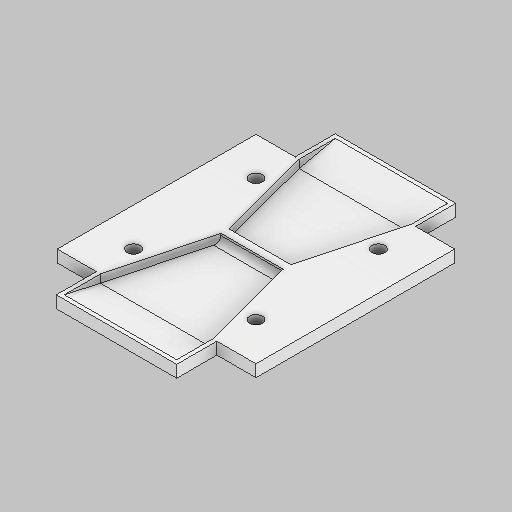
# Autodesk Inventor part: Part4
Saved by Autodesk Inventor 2025.2 (Build 292293000, 293)
## iProperties
Created: 2025-03-19
Part Number: Part4
Material: PC/ABS Plastic
Document SubType Name: Modeling
Designer: joaki
Density: 1.1 g/cm^3
Appearance: Smooth - White
Mass: 7.14549 g
Surface Area: 71.5604 cm^2
Volume: 6.4959 cm^3
Author: joaki
Autodesk Inventor part; units mm, degrees
ref_plane "YZ Plane" through (0, 0, 0) normal (1, 0, 0) x (0, 1, 0)
ref_plane "XZ Plane" through (0, 0, 0) normal (0, 1, 0) x (-1, 0, 0)
ref_plane "XY Plane" through (0, 0, 0) normal (0, 0, 1) x (1, 0, 0)
sketch "Sketch1" plane through (0, 0, 0) normal (0, 1, 0) x (-1, 0, 0)
  line L0 (25.2706, 24.6953) -> (-24.2294, 24.6953)
  line L1 (-24.2294, 24.6953) -> (-24.2294, -24.8047)
  line L2 (-24.2294, -24.8047) -> (25.2706, -24.8047)
  line L3 (25.2706, -24.8047) -> (25.2706, 24.6953)
  circle A0 centre (15.7706, 15.1953) radius 1.6
  circle A1 centre (15.7706, -15.3047) radius 1.6
  circle A2 centre (-14.7294, 15.1953) radius 1.6
  circle A3 centre (-14.7294, -15.3047) radius 1.6
  dimension "d17" = 49.5
  dimension "d18" = 49.5
  dimension "d19" = 3.2
  dimension "d20" = 3.2
  dimension "d21" = 30.5
  dimension "d22" = 9.5
  dimension "d23" = 9.5
  dimension "d24" = 9.5
  dimension "d25" = 9.5
  dimension "d26" = 3.2
  dimension "d27" = 3.2
  dimension "d28" = 30.5
  dimension "d29" = 30.5
  dimension "d30" = 30.5
  dimension "d31" = 9.5
  dimension "d32" = 9.5
  dimension "d33" = 9.5
  dimension "d34" = 9.5
  constraints: 8 end point, 4 centre point, 2 parallel, 1 horizontal, 1 perpendicular
  measures "d17" distance of L1.end L2.end
  measures "d18" distance of L2.end L0.start
  measures "d19" diameter of A0
  measures "d20" diameter of A1
  measures "d21" distance of A1.centre A0.centre
  measures "d22" distance from line of L3 A0.centre
  measures "d23" distance from line of L0 A0.centre
  measures "d24" distance from line of L3 A1.centre
  measures "d25" distance from line of L2 A1.centre
  measures "d26" diameter of A2
  measures "d27" diameter of A3
  measures "d28" distance of A3.centre A1.centre
  measures "d29" distance of A3.centre A2.centre
  measures "d30" distance of A0.centre A2.centre
  measures "d31" distance from line of L1 A3.centre
  measures "d32" distance from line of L0 A2.centre
  measures "d33" distance from line of L1 A2.centre
  measures "d34" distance from line of L2 A3.centre
extrude "Extrusion1" add sketch "Sketch1" along normal blind 3
sketch "Sketch2" plane through (0, 3, 0) normal (0, 1, 0) x (1, 0, 0)
  line L0 (-25.2706, -24.6953) -> (24.2294, -24.6953) projected
  line L1 (-0.5206, -24.6953) -> (-0.5206, 24.8047)
  line L2 (24.2294, 24.8047) -> (-25.2706, 24.8047) projected
  line L3 (-0.5206, -24.6953) -> (-15.5206, -24.6953)
  line L4 (-15.5206, -24.6953) -> (-15.5206, -34.6953)
  line L5 (-15.5206, -34.6953) -> (14.4794, -34.6953)
  line L6 (14.4794, -34.6953) -> (14.4794, -24.6953)
  line L7 (14.4794, -24.6953) -> (-0.5206, -24.6953)
  line L8 (-0.5206, 24.8047) -> (-15.5206, 24.8047)
  line L9 (-15.5206, 24.8047) -> (-15.5206, 34.8047)
  line L10 (-15.5206, 34.8047) -> (14.4794, 34.8047)
  line L11 (14.4794, 34.8047) -> (14.4794, 24.8047)
  line L12 (-0.5206, 24.8047) -> (14.4794, 24.8047)
  point P0 (0, 0)
  dimension "d37" = 15
  dimension "d38" = 10
  dimension "d39" = 30
  dimension "d40" = 15
  dimension "d41" = 10
  dimension "d42" = 30
  constraints: 22 end point, 7 perpendicular, 4 point on line, 2 midpoint, 1 collinear
  measures "d37" distance of L1.start L3.end
  measures "d38" distance of L3.end L4.end
  measures "d39" distance of L4.end L5.end
  measures "d40" distance of L1.end L8.end
  measures "d41" distance of L8.end L9.end
  measures "d42" distance of L9.end L10.end
extrude "Extrusion2" add sketch "Sketch2" against normal blind 3
sketch "Sketch3" plane through (0, 3, 0) normal (0, 1, 0) x (1, 0, 0)
  line L0 (-15.5206, -34.6953) -> (14.4794, -34.6953) projected
  line L1 (-0.5206, -34.6953) -> (-0.5206, 34.8047)
  line L2 (-15.5206, 34.8047) -> (14.4794, 34.8047) projected
  line L3 (-0.5206, -34.6953) -> (-0.5206, -33.6953)
  line L4 (-0.5206, -33.6953) -> (-14.5206, -33.6953)
  line L5 (-14.5206, -33.6953) -> (-14.5206, -24.6953)
  line L6 (-0.5206, -33.6953) -> (13.4794, -33.6953)
  line L7 (13.4794, -33.6953) -> (13.4794, -24.6953)
  line L8 (-0.5206, 34.8047) -> (-0.5206, 33.8047)
  line L9 (-0.5206, 33.8047) -> (-14.5206, 33.8047)
  line L10 (-14.5206, 33.8047) -> (-14.5206, 24.8047)
  line L11 (-0.5206, 33.8047) -> (13.4794, 33.8047)
  line L12 (13.4794, 33.8047) -> (13.4794, 24.8047)
  circle A0 centre (-0.5206, 0.0547) radius 7.5
  line L13 (-14.5206, -24.6953) -> (-8.0206, 0.0547)
  line L14 (-14.5206, 24.8047) -> (-8.0206, 0.0547)
  line L15 (13.4794, -24.6953) -> (6.9794, 0.0547)
  line L16 (13.4794, 24.8047) -> (6.9794, 0.0547)
  point P0 (0, 0)
  dimension "d45" = 1
  dimension "d46" = 14
  dimension "d47" = 14
  dimension "d48" = 1
  dimension "d49" = 14
  dimension "d50" = 14
  dimension "d51" = 15
  constraints: 30 end point, 6 perpendicular, 3 midpoint, 2 horizontal, 2 point on circle, 2 point on line, 1 centre point
  measures "d45" distance of L1.start L3.end
  measures "d46" distance of L3.end L4.end
  measures "d47" distance of L3.end L6.end
  measures "d48" distance of L1.end L8.end
  measures "d49" distance of L8.end L9.end
  measures "d50" distance of L8.end L11.end
  measures "d51" diameter of A0
extrude "Extrusion3" cut sketch "Sketch3" against normal blind 2
sketch "Sketch4" plane through (0, 1, 0) normal (0, 1, 0) x (1, 0, 0)
  point P0 (0, 0)
sketch "Sketch5" plane through (0, 1, 0) normal (0, 1, 0) x (1, 0, 0)
  line L0 (-14.5206, -24.6953) -> (-8.0206, 0.0547) projected
  line L1 (6.9794, 0.0547) -> (13.4794, -24.6953) projected
  line L2 (-8.0206, 0.0547) -> (6.9794, 0.0547)
  line L3 (-8.0206, 0.0547) -> (-8.2747, 1.0219)
  line L4 (-8.0206, 0.0547) -> (-14.5206, 24.8047) projected
  line L5 (-8.0206, 0.0547) -> (-8.2747, -0.9125)
  line L6 (13.4794, 24.8047) -> (6.9794, 0.0547) projected
  line L7 (6.9794, 0.0547) -> (7.2334, 1.0219)
  line L8 (6.9794, 0.0547) -> (7.2334, -0.9125)
  line L9 (7.2334, -0.9125) -> (-8.2747, -0.9125)
  line L10 (-8.2747, 1.0219) -> (7.2334, 1.0219)
  point P0 (0, 0)
  dimension "d56" = 1
  dimension "d57" = 1
  dimension "d58" = 1
  dimension "d59" = 1
  constraints: 14 end point, 4 point on line, 1 horizontal
  measures "d56" distance of L0.end L3.end
  measures "d57" distance of L0.end L5.end
  measures "d58" distance of L1.start L7.end
  measures "d59" distance of L1.start L8.end
extrude "Extrusion4" add sketch "Sketch5" along normal blind 2
fillet "Face Fillet3" radius 1.5 1 edges at (-0.5206, 1, -1.0219)
fillet "Face Fillet4" radius 1.5 1 edges at (-0.5206, 1, 0.9125)
sketch "Sketch6" plane through (-14.5206, 3, -24.8047) normal (1, 0, 0) x (0, 0, -1)
  line L0 (-22.2828, -2) -> (0, -2) projected
  line L1 (9, 0) -> (9, -2) projected
  line L2 (0, -2) -> (9, -2)
  line L3 (9, -2) -> (9, 0)
  line L4 (9, 0) -> (0, -2)
  line L5 (-58.5, 0) -> (-49.5, 0) projected
  line L6 (-58.5, 0) -> (-58.5, -2)
  line L7 (-58.5, -2) -> (-49.5, -2)
  line L8 (-49.5, -2) -> (-58.5, 0)
  point P0 (-24.8047, -3)
  constraints: 12 end point, 2 perpendicular, 1 horizontal, 1 vertical
extrude "Extrusion5" add sketch "Sketch6" along normal blind 28.9875
body "Solid1"
